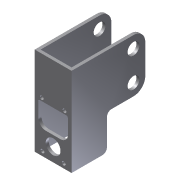
# Autodesk Inventor part: JointC3
Saved by Autodesk Inventor 2011 SP1 (Build 150282100, 282)
## iProperties
Created: 2012-10-16
Part Number: JointC3
Document SubType Name: Modeling
Designer: arihon
Density: 1 g/cm^3
Author: arihon
Autodesk Inventor part; units mm, degrees
ref_plane "YZ Plane" through (0, 0, 0) normal (1, 0, 0) x (0, 1, 0)
ref_plane "XZ Plane" through (0, 0, 0) normal (0, 1, 0) x (-1, 0, 0)
ref_plane "XY Plane" through (0, 0, 0) normal (0, 0, 1) x (1, 0, 0)
sketch "スケッチ1" plane through (0, 0, 0) normal (0, 0, 1) x (1, 0, 0)
  line L0 (-12.5, 25) -> (12.5, 25)
  line L1 (12.5, 25) -> (12.5, -25)
  line L2 (12.5, -25) -> (-12.5, -25)
  line L3 (-12.5, -25) -> (-12.5, 25)
  line L4 (-10.5, 25) -> (10.5, 25)
  line L5 (10.5, 25) -> (10.5, -23)
  line L6 (10.5, -23) -> (-10.5, -23)
  line L7 (-10.5, -23) -> (-10.5, 25)
  point P0 (0, 0)
  dimension "d0" = 25
  dimension "d1" = 50
  dimension "d2" = 25
  dimension "d3" = 12.5
  dimension "d4" = 2
  dimension "d5" = 2
  dimension "d6" = 2
  constraints: 16 end point, 4 parallel, 2 horizontal, 2 perpendicular, 1 point on line
  measures "d0" distance of L0.start L0.end
  measures "d1" distance of L2.end L0.start
  measures "d2" distance from line of L0 point (0, 0)
  measures "d3" distance from line of L3 point (0, 0)
  measures "d4" distance between parallel lines of L3 L7
  measures "d5" distance between parallel lines of L1 L5
  measures "d6" distance between parallel lines of L2 L6
extrude "押し出し1" add sketch "スケッチ1" along normal blind 60 contours L0 L7 L6 L5 L1 L2 L3
sketch "スケッチ2" plane through (12.5, -25, 0) normal (1, 0, 0) x (0, 0, -1)
  line L0 (0, 50) -> (-60, 50) projected
  line L1 (-30, 50) -> (-30, 0)
  line L2 (0, 0) -> (-60, 0) projected
  line L3 (-60, 50) -> (-60, 0) projected
  point P0 (0, 25)
  point P1 (-52, 42)
  point P2 (-32, 42)
  dimension "d11" = 8
  dimension "d12" = 8
  dimension "d76" = 8
  dimension "d84" = 20
  constraints: 2 end point, 2 midpoint
  measures "d11" distance from line of point (-32, 42) L0
  measures "d12" distance from line of L0 point (-52, 42)
  measures "d76" distance from line of L3 point (-52, 42)
  measures "d84" distance of point (-52, 42) point (-32, 42)
hole "Hole1" at (12.5, 17, 52) at (12.5, 17, 32) direction (-1, 0, 0) diameter 8 end through all
sketch "スケッチ5" plane through (-12.5, -25, 0) normal (0, -1, 0) x (1, 0, 0)
  line L0 (25, 60) -> (0, 60) projected
  line L1 (25, 0) -> (25, 60) projected
  line L2 (12.5, 60) -> (12.5, 0)
  line L3 (0, 0) -> (25, 0) projected
  point P0 (4.8, 34.096)
  point P1 (5.3, 2.996)
  point P2 (19.7, 3)
  point P3 (20.2, 34.1)
  dimension "d46" = 14.4
  dimension "d47" = 15.4
  dimension "d48" = 31.1
  dimension "d50" = 15.4
  dimension "d51" = 14.4
  dimension "d52" = 31.1
  dimension "d53" = 3
  constraints: 2 end point, 1 midpoint, 1 parallel
  measures "d46" distance of point (19.7, 3) point (5.3, 2.996)
  measures "d47" distance of point (20.2, 34.1) point (4.8, 34.096)
  measures "d48" vertical distance of point (19.7, 3) point (20.2, 34.1)
  measures "d50" diameter of point (20.2, 34.1) L2
  measures "d51" diameter of point (19.7, 3) L2
  measures "d52" vertical distance of point (5.3, 2.996) point (4.8, 34.096)
  measures "d53" distance from line of L3 point (19.7, 3)
hole "Hole3" at (-7.7, -25, 34.096) at (-7.2, -25, 2.996) at (7.2, -25, 3) at (7.7, -25, 34.1) direction (0, 1, 0) diameter 2.5 end through all
sketch "スケッチ6" plane through (-12.5, -25, 0) normal (0, -1, 0) x (1, 0, 0)
  circle A0 centre (5.3, 2.996) radius 1.25 projected
  point P0 (12.5, 0)
  point P1 (12.5, 9.196)
  dimension "d54" = 7.2
  dimension "d55" = 6.2
  measures "d54" horizontal distance of point (12.5, 9.196) A0.centre
  measures "d55" vertical distance of A0.centre point (12.5, 9.196)
hole "Hole4" at (0, -25, 9.196) direction (0, 1, 0) diameter 10 depth 8 tip angle 118
sketch "スケッチ7" plane through (-12.5, -25, 0) normal (0, -1, 0) x (1, 0, 0)
  circle A0 centre (4.8, 34.096) radius 1.25 projected
  line L0 (25, 60) -> (0, 60) projected
  line L1 (0, 0) -> (25, 0) projected
  line L2 (2.5, 32.096) -> (22.5, 32.096)
  line L3 (22.5, 32.096) -> (22.5, 16.096)
  line L4 (22.5, 16.096) -> (2.5, 16.096)
  line L5 (2.5, 16.096) -> (2.5, 32.096)
  line L6 (12.5, 60) -> (12.5, 0)
  dimension "d63" = 16
  dimension "d64" = 20
  dimension "d65" = 20
  dimension "d66" = 2
  constraints: 10 end point, 2 parallel, 2 perpendicular, 1 horizontal, 1 midpoint
  measures "d63" distance of L4.end L2.start
  measures "d64" distance of L2.start L2.end
  measures "d65" diameter of L5 L6
  measures "d66" distance from line of L2 A0.centre
extrude "押し出し3" cut sketch "スケッチ7" against normal through all contours L2 L6 L4 L5 | L2 L3 L4 L6
fillet "フィレット3" radius 5 2 edges at (-10, -24, 16.096) (10, -24, 16.096)
fillet "フィレット4" radius 1 2 edges at (-10, -24, 32.096) (10, -24, 32.096)
sketch "スケッチ9" plane through (12.5, -25, 0) normal (1, 0, 0) x (0, 0, -1)
  circle A0 centre (-32, 42) radius 4 projected
  line L0 (0, 50) -> (-24, 50)
  line L1 (-24, 50) -> (-24, 24)
  line L2 (-24, 24) -> (0, 24)
  line L3 (0, 24) -> (0, 50)
  line L4 (0, 2) -> (-60, 2) projected
  point P0 (0, 25)
  dimension "d77" = 8
  dimension "d78" = 22
  constraints: 8 end point, 2 parallel, 1 horizontal, 1 perpendicular
  measures "d77" distance from line of L1 A0.centre
  measures "d78" distance between parallel lines of L4 L2
extrude "押し出し5" cut sketch "スケッチ9" against normal through all contours L3 L2 L1 L0
fillet "フィレット5" radius 3 2 edges at (11.5, -1, 24) (-11.5, -1, 24)
fillet "フィレット6" radius 8 4 edges at (-11.5, 25, 60) (11.5, 25, 60) (11.5, 25, 24) (-11.5, 25, 24)
fillet "フィレット7" radius 3 2 edges at (11.5, -1, 0) (-11.5, -1, 0)
equation "\"d1\" = 2 * d0"
equation "\"d2\" = 0.5 * d1"
equation "\"d3\" = 0.5 * d0"
equation "\"d4\" = d5"
equation "\"d6\" = d5"
equation "\"d12\" = d11"
equation "\"d76\" = d11"
equation "\"d50\" = d47"
equation "\"d51\" = d46"
equation "\"d52\" = d48"
equation "\"d65\" = d64"
